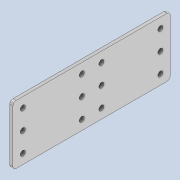
# Autodesk Inventor part: 3x4 2020 Extrusion Gusset Connector
Saved by Autodesk Inventor 2022 (Build 260153000, 153)
## iProperties
Created: 2021-11-27
Part Number: 3x4 2020 Extrusion Gusset Connector
Material: Generic
Document SubType Name: Modeling
Designer: Coy
Density: 1 g/cm^3
Appearance: Machined - Aluminum
Author: Coy
Autodesk Inventor part; units mm, degrees
ref_plane "YZ Plane" through (0, 0, 0) normal (1, 0, 0) x (0, 1, 0)
ref_plane "XZ Plane" through (0, 0, 0) normal (0, 1, 0) x (-1, 0, 0)
ref_plane "XY Plane" through (0, 0, 0) normal (0, 0, 1) x (1, 0, 0)
sketch "Sketch1" plane through (0, 0, 0) normal (1, 0, 0) x (0, 1, 0)
  line L0 (0, 0) -> (60, 0)
  line L1 (60, 0) -> (60, 160)
  line L2 (60, 160) -> (0, 160)
  line L3 (0, 160) -> (0, 0)
  line L4 (50, 150) -> (10, 150) construction
  line L5 (10, 150) -> (10, 10) construction
  line L6 (10, 10) -> (50, 10) construction
  line L7 (50, 10) -> (50, 150) construction
  line L8 (50, 80) -> (10, 80) construction
  line L9 (50, 70) -> (10, 70) construction
  line L10 (50, 90) -> (10, 90) construction
  line L11 (30, 150) -> (30, 10) construction
  circle A0 centre (50, 150) radius 2.6
  circle A1 centre (30, 150) radius 2.6
  circle A2 centre (10, 150) radius 2.6
  circle A3 centre (30, 90) radius 2.6
  circle A4 centre (50, 90) radius 2.6
  circle A5 centre (10, 90) radius 2.6
  circle A6 centre (10, 70) radius 2.6
  circle A7 centre (30, 70) radius 2.6
  circle A8 centre (50, 70) radius 2.6
  circle A9 centre (50, 10) radius 2.6
  circle A10 centre (30, 10) radius 2.6
  circle A11 centre (10, 10) radius 2.6
  dimension "d0" = 60
  dimension "d1" = 160
  dimension "d2" = 10
  dimension "d3" = 10
  dimension "d4" = 10
  dimension "d5" = 10
  dimension "d6" = 10
  dimension "d7" = 10
  dimension "d8" = 5.2
  dimension "d9" = 5.2
  dimension "d10" = 5.2
  dimension "d11" = 5.2
  dimension "d12" = 5.2
  dimension "d13" = 5.2
  dimension "d14" = 5.2
  dimension "d15" = 5.2
  dimension "d16" = 5.2
  dimension "d17" = 5.2
  dimension "d18" = 5.2
  dimension "d19" = 5.2
  constraints: 24 end point, 12 centre point, 10 coincident, 6 midpoint, 6 parallel, 6 point on line, 2 horizontal, 2 perpendicular
  measures "d0" distance of L2.end L1.end
  measures "d1" distance of L1.end L0.end
  measures "d2" distance between parallel lines of L2 L4
  measures "d3" distance between parallel lines of L0 L6
  measures "d4" distance between parallel lines of L1 L7
  measures "d5" distance between parallel lines of L3 L5
  measures "d6" distance between parallel lines of L8 L9
  measures "d7" distance between parallel lines of L8 L10
  measures "d8" diameter of A0
  measures "d9" diameter of A1
  measures "d10" diameter of A2
  measures "d11" diameter of A4
  measures "d12" diameter of A3
  measures "d13" diameter of A5
  measures "d14" diameter of A8
  measures "d15" diameter of A7
  measures "d16" diameter of A6
  measures "d17" diameter of A11
  measures "d18" diameter of A10
  measures "d19" diameter of A9
extrude "Extrusion1" add sketch "Sketch1" along normal blind 3.175
fillet "Fillet1" radius 3.175 4 edges at (1.5875, 60, 160) (1.5875, 0, 160) (1.5875, 60, 0) (1.5875, 0, 0)
equation "\"d3\" = d2"
equation "\"d4\" = d2"
equation "\"d5\" = d2"
equation "\"d9\" = d8"
equation "\"d10\" = d8"
equation "\"d11\" = d8"
equation "\"d12\" = d8"
equation "\"d13\" = d8"
equation "\"d14\" = d8"
equation "\"d15\" = d8"
equation "\"d16\" = d8"
equation "\"d17\" = d8"
equation "\"d18\" = d8"
equation "\"d19\" = d8"
body "Solid1"
